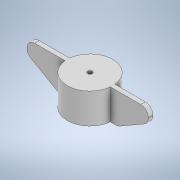
# Autodesk Inventor part: top_propeller
Saved by Autodesk Inventor 2021 (Build 250183000, 183)
## iProperties
Created: 2023-05-04
Part Number: top_propeller
Material: Generic
Document SubType Name: Modeling
Designer: assman
Density: 1 g/cm^3
Appearance: Default
Author: assman
Autodesk Inventor part; units mm, degrees
ref_plane "YZ Plane" through (0, 0, 0) normal (1, 0, 0) x (0, 1, 0)
ref_plane "XZ Plane" through (0, 0, 0) normal (0, 1, 0) x (-1, 0, 0)
ref_plane "XY Plane" through (0, 0, 0) normal (0, 0, 1) x (1, 0, 0)
sketch "Sketch1" plane through (0, 0, 0) normal (0, 1, 0) x (-1, 0, 0)
  line L0 (15, 0) -> (40, 0) construction
  line L1 (-15, 0) -> (-40, 0) construction
  line L2 (14.9248, -1.5) -> (39.9719, -1.5)
  line L3 (14.9248, 1.5) -> (39.9719, 1.5)
  line L4 (-14.9248, -1.5) -> (-39.9719, -1.5)
  line L5 (-14.9248, 1.5) -> (-39.9719, 1.5)
  arc A0 (-39.9719, 1.5) -> (-39.9719, -1.5) centre (0, 0) ccw
  arc A1 (39.9719, -1.5) -> (39.9719, 1.5) centre (0, 0) ccw
  arc A2 (14.9248, 1.5) -> (-14.9248, 1.5) centre (0, 0) ccw
  arc A3 (-14.9248, -1.5) -> (14.9248, -1.5) centre (0, 0) ccw
  dimension "d2" = 1.5
  dimension "d3" = 1.5
  dimension "d4" = 1.5
  dimension "d5" = 1.5
  constraints: 12 end point, 10 point on circle, 4 centre point, 4 parallel, 2 coincident, 2 point on line, 1 horizontal
  measures "d2" distance between parallel lines of L0 L2
  measures "d3" distance between parallel lines of L0 L3
  measures "d4" distance between parallel lines of L1 L4
  measures "d5" distance between parallel lines of L1 L5
extrude "Extrusion1" add sketch "Sketch1" along normal blind 20
fillet "Fillet1" radius 5 2 edges at (40, 20, 0) (-40, 20, 0)
chamfer "Chamfer1" distance 20 angle 30 1 edges at (-40, 0, 0) measured on face at (-39.5, 0, 0)
chamfer "Chamfer2" distance 20 angle 30 1 edges at (40, 0, 0) measured on face at (39.5, 0, 0)
fillet "Fillet2" radius 5 2 edges at (40, 11.547, 0) (-40, 11.547, 0)
fillet "Fillet3" radius 5 2 edges at (20, 0, 0) (-20, 0, 0)
sketch "Sketch3" plane through (0, 20, 0) normal (0, 1, 0) x (1, 0, 0)
  arc A0 (-34.9678, 1.5) -> (-34.9678, -1.5) centre (0, 0) ccw construction
  line L0 (-34.9678, -1.5) -> (-14.9248, -1.5) construction
  arc A1 (-14.9248, -1.5) -> (14.9248, -1.5) centre (0, 0) ccw construction
  line L1 (14.9248, -1.5) -> (34.9678, -1.5) construction
  arc A2 (34.9678, -1.5) -> (34.9678, 1.5) centre (0, 0) ccw construction
  line L2 (34.9678, 1.5) -> (14.9248, 1.5) construction
  arc A3 (14.9248, 1.5) -> (-14.9248, 1.5) centre (0, 0) ccw construction
  line L3 (-14.9248, 1.5) -> (-34.9678, 1.5) construction
  circle A4 centre (0, 0) radius 1.5
  dimension "d36" = 3
  constraints: 1 centre point, 1 coincident
  measures "d36" diameter of A4
extrude "Extrusion2" cut sketch "Sketch3" against normal through all
equation "\"d2\" = 0.5 * blade_width"
equation "\"d3\" = 0.5 * blade_width"
equation "\"d4\" = 0.5 * blade_width"
equation "\"d5\" = 0.5 * blade_width"
equation "\"blade_width\" = 3"
equation "\"d21\" = 0"
equation "\"d22\" = 5"
equation "\"d23\" = 3"
equation "\"d24\" = 5"
equation "\"d25\" = 0"
equation "\"d8\" = 0.5 * blade_width"
equation "\"d9\" = 0.5 * blade_width"
equation "\"d10\" = 0.5 * blade_width"
equation "\"d11\" = 0.5 * blade_width"
equation "\"d12\" = 0.5 * blade_width"
equation "\"d13\" = 0.5 * blade_width"
equation "\"d14\" = 0.5 * blade_width"
equation "\"d15\" = 0.5 * blade_width"
equation "\"d16\" = 0.5 * blade_width"
equation "\"d17\" = 0.5 * blade_width"
equation "\"d18\" = 0.5 * blade_width"
equation "\"d19\" = 0.5 * blade_width"
body "Solid1"
